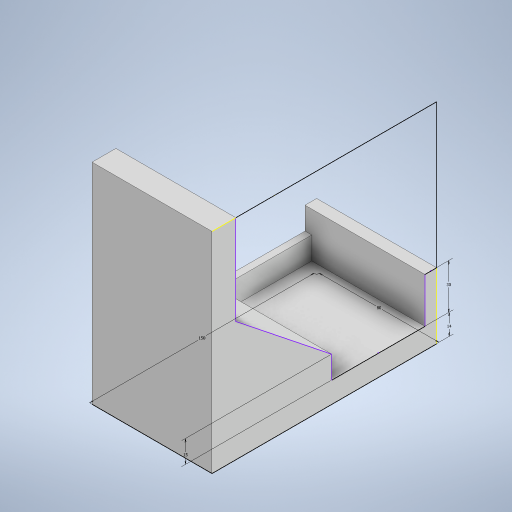
# Autodesk Inventor part: Left
Saved by Autodesk Inventor 2023.2 (Build 272271030, 271C)
## iProperties
Created: 2024-03-06
Part Number: Left
Material: Generic
Document SubType Name: Modeling
Designer: ryanv
Density: 1 g/cm^3
Appearance: Default
Author: ryanv
Autodesk Inventor part; units mm, degrees
ref_plane "YZ Plane" through (0, 0, 0) normal (1, 0, 0) x (0, 1, 0)
ref_plane "XZ Plane" through (0, 0, 0) normal (0, 1, 0) x (-1, 0, 0)
ref_plane "XY Plane" through (0, 0, 0) normal (0, 0, 1) x (1, 0, 0)
sketch "Sketch1" plane through (0, 0, 0) normal (0, 1, 0) x (-1, 0, 0)
  line L0 (0, 0) -> (80, 0)
  line L1 (80, 0) -> (80, -150)
  line L2 (80, -150) -> (0, -150)
  line L3 (0, -150) -> (0, 0)
  dimension "d0" = 80
  dimension "d1" = 150
  constraints: 8 end point, 2 parallel, 1 horizontal, 1 perpendicular
  measures "d0" distance of L1.end L2.end
  measures "d1" distance of L0.end L1.end
extrude "Extrusion1" add sketch "Sketch1" along normal blind 140
sketch "Sketch2" plane through (0, 0, 0) normal (1, 0, 0) x (0, 0, -1)
  line L0 (150, 140) -> (0, 140) projected
  line L1 (15.8986, 80) -> (79.9832, 29)
  line L2 (79.9832, 29) -> (79.9832, 14)
  line L3 (79.9832, 14) -> (142.2187, 14)
  line L4 (142.2187, 14) -> (142.2187, 44)
  line L5 (142.2187, 44) -> (150, 44)
  line L6 (150, 0) -> (150, 140) projected
  line L7 (150, 44) -> (150, 140)
  line L8 (150, 140) -> (61.0962, 140)
  line L9 (15.8986, 100) -> (15.8986, 80)
  line L10 (0, 0) -> (150, 0) projected
  line L11 (61.0962, 140) -> (15.8986, 140)
  line L12 (15.8986, 100) -> (15.8986, 140)
  point P0 (146.1093, 44)
  point P1 (111.101, 14)
  dimension "d7" = 15
  dimension "d8" = 30
  dimension "d9" = 14
  constraints: 20 end point, 7 perpendicular, 2 midpoint, 2 point on line
  measures "d7" distance from line of L3 L1.end
  measures "d8" distance from line of L3 point (146.109, 44)
  measures "d9" distance from line of L10 point (111.101, 14)
extrude "Extrusion2" cut sketch "Sketch2" against normal blind 140
sketch "Sketch6" plane through (0, 14, -79.9832) normal (0, 1, 0) x (1, 0, 0)
  line L0 (0, 62.2355) -> (-80, 62.2355) projected
  line L1 (0, 0) -> (-80, 0) projected
  line L2 (-80, 62.2355) -> (-75.5003, 62.2355)
  line L3 (-75.5003, 62.2355) -> (-75.5003, 0)
  line L4 (-75.5003, 0) -> (-80, 0)
  line L5 (-80, 0) -> (-80, 62.2355)
  point P0 (0, -79.9832)
  constraints: 8 end point, 2 parallel, 1 horizontal, 1 perpendicular, 1 point on line
extrude "Extrusion6" add sketch "Sketch6" along normal blind 15
body "Solid1"
